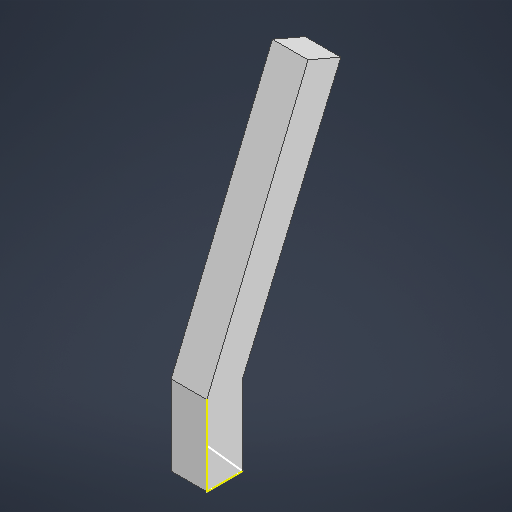
# Autodesk Inventor part: Arm_Servo_Cone
Saved by Autodesk Inventor 2026.1 (Build 301233000, 233)
## iProperties
Created: 2025-09-01
Part Number: Arm_Servo_Cone
Material: Generic
Document SubType Name: Modeling
Designer: junha
Density: 1 g/cm^3
Appearance: Default
Author: junha
Autodesk Inventor part; units mm, degrees
ref_plane "YZ Plane" through (0, 0, 0) normal (1, 0, 0) x (0, 1, 0)
ref_plane "XZ Plane" through (0, 0, 0) normal (0, 1, 0) x (-1, 0, 0)
ref_plane "XY Plane" through (0, 0, 0) normal (0, 0, 1) x (1, 0, 0)
sketch "Sketch1" plane through (0, 0, 0) normal (1, 0, 0) x (0, 1, 0)
  line L0 (0, 0) -> (0, -10)
  line L1 (0, -10) -> (22.36, -10)
  line L2 (22.36, -10) -> (86.7001, -37.5744)
  line L3 (22.36, -10) -> (92.36, -10) construction
  line L4 (86.7001, -37.5744) -> (90.6393, -28.3829)
  line L5 (0, 0) -> (22.36, 0)
  line L6 (22.36, 0) -> (90.6393, -28.3829)
  dimension "d0" = 10
  dimension "d1" = 22.36
  dimension "d2" = 70
  dimension "d3" = 23.199
  dimension "d4" = 10
  constraints: 14 end point, 2 horizontal, 2 perpendicular, 1 equal length, 1 vertical
  measures "d0" distance of L0.start L0.end
  measures "d1" distance of L0.end L1.end
  measures "d2" distance of L1.end L2.end
  measures "d3" angle of L2 L3
  measures "d4" distance of L2.end L4.end
extrude "Extrusion1" add sketch "Sketch1" along normal blind 10
sketch "Sketch2" plane through (10, 0, 0) normal (1, 0, 0) x (0, 0, -1)
  line L0 (0, 0) -> (10, 0) projected
  line L1 (10, 0) -> (0, 11.18)
  line L2 (0, 22.36) -> (0, 0) projected
  line L3 (0, 11.18) -> (0, 0)
  line L4 (0, 0) -> (10, 0)
  constraints: 6 end point, 1 collinear, 1 midpoint, 1 perpendicular
body "Solid1"
